Autodesk Fusion 360 part; units mm, degrees
(part 2 of 2)
  line L173 (-36.9567, -45.6022) -> (-30.8108, -39.3141)
  line L174 (-30.8108, -39.3141) -> (-19.5682, -39.395)
  line L175 (-19.5682, -39.395) -> (-13.294, -45.587)
  line L176 (-13.294, -45.587) -> (-13.294, -50.7432)
  spline S48 degree 3 poles (-13.294, -50.7432) (-9.5914, -50.0109) (-5.9637, -48.9591) (-2.8564, -47.6206) knots 0 0 0 0 1 1 1 1
  line L177 (-2.8564, -47.6206) -> (-2.8564, -41.2087)
  line L178 (-2.8564, -41.2087) -> (-15.2543, -28.9993)
  line L179 (-15.2543, -28.9993) -> (-35.1117, -28.845)
  line L180 (-35.1117, -28.845) -> (-47.4023, -41.267)
  line L181 (-47.4023, -41.267) -> (-47.4037, -47.6301)
  spline S49 degree 3 poles (-47.4037, -47.6301) (-44.1351, -49.0146) (-40.8088, -50.0214) (-36.9662, -50.7771) knots 0 0 0 0 1 1 1 1
  line L182 (-36.9662, -50.7771) -> (-36.9659, -50.7766)
extrude "Extrude11" cut sketch "Sketch7" against normal blind 1 contours L21 L22 L23 L24 L25 L26 L27 L28 L29 L30 L31 L32 L33 L34 L35 L36 L37 L38 L39 L40 L41 L42 | L44 S5 L45 S6 L46 S7 L47 S8 | S9 L49 L50 L51 S10 L52 L53 L54 | L56 L57 S11 L58 L59 L60 S12 L61 L62 S13 | S14 L65 S15 L66 | S16 L67 L68 L69 S17 L70 S18 L71 S19 L72 S20 L73 | L76 S21 L77 S22 L78 S23 L79 S24 | L94 S26 L95 S27 L96 S28 L97 S29 L98 S30 L99 S31 | S32 L101 L102 L103 S33 L104 L105 L106 | L113 L114 S34 L115 S35 L116 L117 L118 L119 L120 S36 L121 S37 L122 L123 L124 L125 | L126 L127 S38 L128 L129 L130 L131 L132 S39 L133 L134 L135 | L137 L138 L139 L140 L141 S40 L142 L143 L144 L145 L146 S41 | S42 L148 S43 L149 L150 L151 L152 L153 S44 L154 S45 L155 L156 L157 L158 L159 | L161 L162 S46 L163 L164 L165 L166 L167 S47 L168 L169 L170 | L172 L173 L174 L175 L176 S48 L177 L178 L179 L180 L181 S49 bodies 1
equation "scale = 0.5" comment "scale"
equation "d2 = ( 0.05 * scale ) * 1 m"
equation "d3 = ( 0.048 * scale ) * 1 m"
equation "d4 = ( 0.048 * scale ) * 1 m"
equation "d5 = ( 0.16 * scale ) * 1 m"
equation "d6 = ( 0.05 * scale ) * 1 m"
equation "d7 = ( 0.048 * scale ) * 1 m"
equation "d8 = ( 0.048 * scale ) * 1 m"
equation "half_gap = 0.001 m"
equation "d10 = half_gap"
equation "d11 = half_gap"
equation "d13 = 0.005 m + half_gap"
equation "gap_depth = 0.005 m"
equation "d15 = -gap_depth"
equation "d39 = ( 0.015 * scale ) * 1 m"
equation "d40 = ( 0.02 * scale ) * 1 m"
equation "d41 = ( 0.0541 * scale ) * 1 m"
equation "d42 = ( -0.0603 * scale ) * 1 m"
equation "d43 = ( 0.0653 * scale ) * 1 m"
equation "d44 = -gap_depth / 2"
equation "d47 = -gap_depth - 0.001 m"
